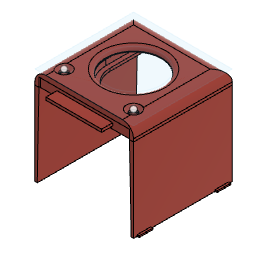
TankHoseMount_v8 (Autodesk Fusion 360 design; units mm, degrees)
Autodesk Fusion 360 part; units mm, degrees
note: some values were not read from the file. Chosen so that the rebuilt part matches the saved one: which face or edge a step refers to. Set by a fixed rule: which sketch regions a step uses.
sketch "Sketch1" plane through (0, 0, 0) normal (0, 0, 1) x (1, 0, 0)
  line L0 (35.5, -35.5) -> (-35.5, -35.5)
  line L1 (-35.5, -35.5) -> (-35.5, 35.5)
  line L2 (-35.5, 35.5) -> (35.5, 35.5)
  line L3 (35.5, 35.5) -> (35.5, -35.5)
  line L4 (35.5, -35.5) -> (-35.5, 35.5) construction
  line L5 (-35.5, -35.5) -> (35.5, 35.5) construction
  circle A0 centre (0, 0) radius 20
  dimension "d1" = 71
  dimension "d2" = 71
  dimension "d3" = 40
  constraint horizontal L0
  constraint perpendicular L0 L1
  constraint parallel L0 L2
  constraint parallel L1 L3
  constraint coincident L4 A0.centre
  constraint coincident L5 A0.centre
  constraint coincident A0.centre origin
  measures "d1" distance of L1.end L2.end
  measures "d2" distance of L0.end L1.end
  measures "d3" diameter of A0
extrude "Extrude1" add sketch "Sketch1" along normal blind 10 makes body 1
sketch "Sketch2" plane through (0, -35.5, 0) normal (0, -1, 0) x (1, 0, 0)
  line L0 (-35.5, 0) -> (35.5, 0)
  line L1 (35.5, 0) -> (35.5, 10)
  line L2 (35.5, 10) -> (-35.5, 10)
  line L3 (-35.5, 10) -> (-35.5, 0)
  line L4 (-32.5, 6.5) -> (32.5, 6.5)
  line L5 (32.5, 6.5) -> (32.5, 0)
  line L6 (32.5, 0) -> (-32.5, 0)
  line L7 (-32.5, 0) -> (-32.5, 6.5)
  dimension "d8" = 6.5
  dimension "d10" = 3
  dimension "d11" = 3
  constraint horizontal L4
  constraint vertical L5
  constraint horizontal L6
  constraint vertical L7
  constraint coincident L0 L5.end
  measures "d8" distance of L4.start L6.end
  measures "d10" distance of L1 L5.end
  measures "d11" distance of L3 L7
extrude "Extrude2" cut sketch "Sketch2" against normal blind 69 contours L0 L4 L5 L6 L7 bodies 1
sketch "Sketch3" plane through (0, 0, 0) normal (0, 0, -1) x (1, 0, 0)
  line L0 (-32.5, -33.5) -> (-32.5, 35.5)
  line L1 (-32.5, 35.5) -> (-35.5, 35.5)
  line L2 (-35.5, 35.5) -> (-35.5, -35.5)
  line L3 (-35.5, -35.5) -> (35.5, -35.5)
  line L4 (35.5, -35.5) -> (35.5, 35.5)
  line L5 (35.5, 35.5) -> (32.5, 35.5)
  line L6 (32.5, 35.5) -> (32.5, -33.5)
  line L7 (32.5, -33.5) -> (-32.5, -33.5)
  line L8 (-35.5, 35.5) -> (-32.5, 35.5)
  line L9 (-32.5, 35.5) -> (-32.5, -35.5)
  line L10 (-32.5, -35.5) -> (-35.5, -35.5)
  line L11 (-35.5, -35.5) -> (-35.5, 35.5)
  line L12 (32.5, 35.5) -> (35.5, 35.5)
  line L13 (35.5, 35.5) -> (35.5, -35.5)
  line L14 (35.5, -35.5) -> (32.5, -35.5)
  line L15 (32.5, -35.5) -> (32.5, 35.5)
  constraint horizontal L8
  constraint vertical L9
  constraint horizontal L10
  constraint vertical L11
  constraint coincident L3 L9.end
  constraint coincident L1.end L2.start
  constraint horizontal L12
  constraint vertical L13
  constraint horizontal L14
  constraint vertical L15
  constraint coincident L3.end L4.start
  constraint coincident L5.end L6.start
ref_plane "WorkPlane1" through (34, 0, -60) normal (0, 0, -1) x (1, 0, 0)
sketch "Sketch4" plane through (34, 0, -60) normal (0, 0, -1) x (1, 0, 0)
  line L0 (-69.5, 35.5) -> (-67.75, 35.5)
  line L1 (-67.75, 35.5) -> (-67.75, -35.5)
  line L2 (-67.75, -35.5) -> (-69.5, -35.5)
  line L3 (-69.5, -35.5) -> (-69.5, 35.5)
  line L4 (1.5, 35.5) -> (-0.25, 35.5)
  line L5 (-0.25, 35.5) -> (-0.25, -35.5)
  line L6 (-0.25, -35.5) -> (1.5, -35.5)
  line L7 (1.5, -35.5) -> (1.5, 35.5)
  point P0 (1.5, 35.5)
  dimension "d13" = 1.75
  dimension "d14" = 71
  dimension "d15" = 1.75
  dimension "d16" = 71
  constraint horizontal L0
  constraint vertical L1
  constraint horizontal L2
  constraint vertical L3
  constraint horizontal L4
  constraint vertical L5
  constraint horizontal L6
  constraint vertical L7
  measures "d13" distance of L0.start L0.end
  measures "d14" distance of L0.start L2.end
  measures "d15" distance of P0 L4.end
  measures "d16" distance of P0 L6.end
ref_plane "WorkPlane2" through (-34, 0, -20) normal (0, 0, -1) x (1, 0, 0)
sketch "Sketch5" plane through (-34, 0, -20) normal (0, 0, -1) x (1, 0, 0)
  line L0 (-1.5, 35.5) -> (1, 35.5)
  line L1 (1, 35.5) -> (1, -35.5)
  line L2 (1, -35.5) -> (-1.5, -35.5)
  line L3 (-1.5, -35.5) -> (-1.5, 35.5)
  line L4 (69.5, 35.5) -> (67, 35.5)
  line L5 (67, 35.5) -> (67, -35.5)
  line L6 (67, -35.5) -> (69.5, -35.5)
  line L7 (69.5, -35.5) -> (69.5, 35.5)
  dimension "d18" = 2.5
  dimension "d19" = 71
  dimension "d20" = 2.5
  dimension "d21" = 71
  constraint horizontal L0
  constraint vertical L1
  constraint horizontal L2
  constraint vertical L3
  constraint horizontal L4
  constraint vertical L5
  constraint horizontal L6
  constraint vertical L7
  measures "d18" distance of L0.start L0.end
  measures "d19" distance of L0.start L2.end
  measures "d20" distance of L4.start L4.end
  measures "d21" distance of L4.start L6.end
loft "Loft1" add profiles "Sketch3", "Sketch5", "Sketch4" section 1 contours L0 L1 L2 L3 L8 L9 L10 L11 section 2 contours L0 L1 L2 L3 section 3 contours L0 L1 L2 L3 bodies 1
loft "Loft2" add profiles "Sketch3", "Sketch5", "Sketch4" section 1 contours L3 L4 L5 L6 L12 L13 L14 L15 section 2 contours L4 L5 L6 L7 section 3 contours L4 L5 L6 L7 bodies 1
sketch "Sketch6" plane through (35.5, 0, 0) normal (1, 0, 0) x (0, 1, 0)
  line L0 (35.5, 0) -> (-35.5, 0)
  line L1 (-35.5, 0) -> (-35.5, -60)
  line L2 (-35.5, -60) -> (35.5, -60)
  line L3 (35.5, -60) -> (35.5, 0)
  line L4 (-33, -60) -> (-23, -60)
  line L5 (-23, -60) -> (-23, -59)
  line L6 (-23, -59) -> (-33, -59)
  line L7 (-33, -59) -> (-33, -60)
  line L8 (23, -60) -> (33, -60)
  line L9 (33, -60) -> (33, -59)
  line L10 (33, -59) -> (23, -59)
  line L11 (23, -59) -> (23, -60)
  line L12 (0, -60) -> (0, -38) construction
  dimension "d22" = 10
  dimension "d23" = 1
  dimension "d24" = 10
  dimension "d25" = 1
  dimension "d27" = 23
  dimension "d28" = 23
  constraint horizontal L4
  constraint vertical L5
  constraint horizontal L6
  constraint vertical L7
  constraint coincident L2 L4.start
  constraint horizontal L8
  constraint vertical L9
  constraint horizontal L10
  constraint vertical L11
  constraint coincident L2 L8.start
  constraint midpoint L2 L12.start
  constraint perpendicular L2 L12
  measures "d22" distance of L4.start L4.end
  measures "d23" distance of L4.start L6.end
  measures "d24" distance of L8.start L8.end
  measures "d25" distance of L8.start L10.end
  measures "d27" distance of L5.end L12
  measures "d28" distance of L10.end L12
sketch "Sketch7" plane through (-35.5, 0, 0) normal (-1, 0, 0) x (0, -1, 0)
  line L0 (35.5, 0) -> (-35.5, 0)
  line L1 (-35.5, 0) -> (-35.5, -60)
  line L2 (-35.5, -60) -> (35.5, -60)
  line L3 (35.5, 0) -> (35.5, -60)
sketch "Sketch8" plane through (-35.5, 0, -30) normal (-1, 0, 0) x (0, -1, 0)
  line L0 (-33, -29) -> (-23, -29)
  line L1 (-23, -29) -> (-23, -30)
  line L2 (-23, -30) -> (-33, -30)
  line L3 (-33, -30) -> (-33, -29)
  line L4 (23, -29) -> (33, -29)
  line L5 (33, -29) -> (33, -30)
  line L6 (33, -30) -> (23, -30)
  line L7 (23, -30) -> (23, -29)
  constraint horizontal L0
  constraint vertical L1
  constraint horizontal L2
  constraint vertical L3
  constraint horizontal L4
  constraint vertical L5
  constraint horizontal L6
  constraint vertical L7
extrude "Extrude3" add sketch "Sketch6" along normal blind 1.5 contours L2 L8 L9 L10 L11 | L2 L4 L5 L6 L7 bodies 1
extrude "Extrude4" add sketch "Sketch8" along normal blind 2 bodies 1
copy_body "Body->Comp1" bodies 1 removing the originals makes body 2 in component "Component"
sketch "Sketch9" plane through (0, 0, 0) normal (0, 0, 1) x (1, 0, 0)
  circle A0 centre (0, 0) radius 17
  line L0 (-32, -35) -> (32, -35)
  line L1 (32, -35) -> (32, 33)
  line L2 (32, 33) -> (-32, 33)
  line L3 (-32, 33) -> (-32, -35)
  line L4 (-17, 0) -> (-17, 33)
  line L5 (17, 0) -> (17, 33)
  circle A1 centre (0, 0) radius 20
  line L6 (-20, 0) -> (-20, 33)
  line L7 (20, 0) -> (20, 33)
  dimension "d33" = 34
  constraint coincident A0.centre A1.centre
  constraint horizontal L0
  constraint vertical L1
  constraint horizontal L2
  constraint vertical L3
  constraint coincident L2 L4.end
  constraint perpendicular L2 L4
  constraint tangent A0 L4
  constraint coincident L2 L5.end
  constraint perpendicular L2 L5
  constraint tangent A0 L5
  constraint coincident A0 L4.start
  constraint coincident A1 L6.start
  constraint coincident L2 L6.end
  constraint tangent A1 L6
  constraint perpendicular L2 L6
  constraint coincident A1 L7.start
  constraint coincident L2 L7.end
  constraint tangent A1 L7
  constraint perpendicular L2 L7
  measures "d33" diameter of A0
extrude "Extrude5" add sketch "Sketch9" along normal blind 6 separate body contours L0 L1 L2 L3 A1 L6 L7 makes body 3
extrude "Extrude6" add sketch "Sketch9" along normal blind 2 contours A0 L4 L5 A1 | L2 L5 A1 L7 | L2 L4 A1 L6 picked at (18.9255, -0.9936) bodies 3
sketch "Sketch10" plane through (0, -35, 0) normal (0, -1, 0) x (1, 0, 0)
  line L0 (-32, 0) -> (32, 0)
  line L1 (32, 0) -> (32, 6)
  line L2 (32, 6) -> (-32, 6)
  line L3 (-32, 6) -> (-32, 0)
  line L4 (20, 4) -> (-20, 4)
  line L5 (-20, 4) -> (-20, 2)
  line L6 (-20, 2) -> (20, 2)
  line L7 (20, 2) -> (20, 4)
  line L8 (20, 4) -> (-20, 2) construction
  line L9 (-20, 4) -> (20, 2) construction
  point P0 (0, 3)
  dimension "d38" = 40
  dimension "d39" = 2
  constraint horizontal L4
  constraint perpendicular L4 L5
  constraint parallel L4 L6
  constraint parallel L5 L7
  constraint coincident L8 P0
  constraint coincident L9 P0
  measures "d38" distance of L5.end L6.end
  measures "d39" distance of L4.end L5.end
extrude "Extrude7" add sketch "Sketch10" along normal blind 8 contours L4 L5 L6 L7 bodies 3
sketch "Sketch11" plane through (0, 0, 10) normal (0, 0, 1) x (-1, 0, 0)
  circle A0 centre (0, 0) radius 20
  line L0 (-35.5, -35.5) -> (35.5, -35.5)
  line L1 (35.5, -35.5) -> (35.5, 35.5)
  line L2 (35.5, 35.5) -> (-35.5, 35.5)
  line L3 (-35.5, 35.5) -> (-35.5, -35.5)
  point P0 (25, 25)
  point P1 (-25, 25)
hole "Hole1" at (-25, -25, 10) at (25, -25, 10) direction (0, 0, -1) diameter 5.8 depth 3.5 tip angle 180 countersink diameter 10.4 countersink angle 90 bodies 2 in component "Component"
hole "Hole1'" at (-25, -25, 10) at (25, -25, 10) direction (0, 0, -1) diameter 5.3 depth 35 tip angle 180 countersink diameter 10.4 countersink angle 90 bodies 3
fillet "Fillet1" radius 8 3 edges at (35.5, 0, 10) (0, 35.5, 10) (-35.5, 0, 10) on bodies 2 in component "Component"
fillet "Fillet2" radius 3 1 edges at (-18.6465, 7.2323, 10) on bodies 2 in component "Component"
copy_body "Body->Comp2" bodies 3 removing the originals makes body 4 in component "Component'"
component "Component" placed x (1, 0, 0) y (0, 1, 0) z (0, 0, 1) at (0, 0, 0)
component "Component'" placed x (1, 0, 0) y (0, 1, 0) z (0, 0, 1) at (0, 0, 0)
